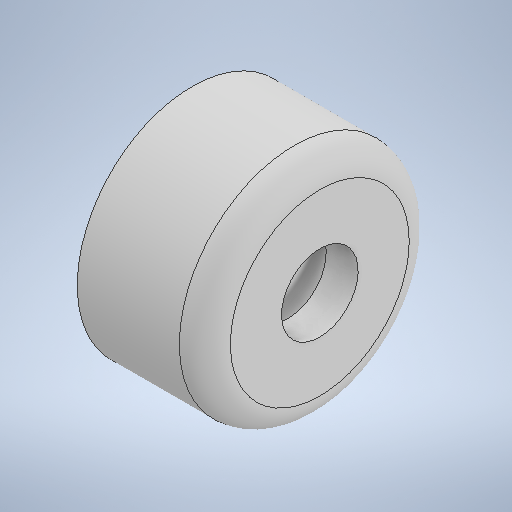
# Autodesk Inventor part: 14.2
Saved by Autodesk Inventor 2025.1 (Build 291241000, 241)
## iProperties
Created: 2024-09-13
Part Number: 14.2
Material: Generisch
Document SubType Name: Modeling
Designer: ffogue
Density: 1 g/cm^3
Appearance: Vorgabe
Author: ffogue
Autodesk Inventor part; units mm, degrees
ref_plane "YZ Plane" through (0, 0, 0) normal (1, 0, 0) x (0, 1, 0)
ref_plane "XZ Plane" through (0, 0, 0) normal (0, 1, 0) x (-1, 0, 0)
ref_plane "XY Plane" through (0, 0, 0) normal (0, 0, 1) x (1, 0, 0)
sketch "Sketch1" plane through (0, 0, 0) normal (0, 0, 1) x (1, 0, 0)
  line L0 (0, 6) -> (0, 9)
  line L1 (0, 9) -> (10, 9)
  line L2 (10, 9) -> (10, 0)
  line L3 (10, 0) -> (0, 0)
  line L4 (0, 6) -> (5.5, 6)
  line L5 (5.5, 6) -> (7.5, 4)
  line L6 (7.5, 4) -> (7.5, 0)
  point P0 (5, 9)
  dimension "d0" = 45
  dimension "d1" = 18
  dimension "d2" = 12
  dimension "d3" = 2.5
  dimension "d4" = 10
  dimension "d5" = 2
  constraints: 14 end point, 4 perpendicular, 1 horizontal, 1 midpoint, 1 point on line, 1 vertical, 1 vertical alignment
  measures "d0" angle of L5 L4
  measures "d1" diameter of point (5, 9) L3
  measures "d2" diameter of L4 L3
  measures "d3" distance between parallel lines of L2 L6
  measures "d4" distance of L0.end L1.end
  measures "d5" distance from line of L5.end L4
revolve "Revolution1" add sketch "Sketch1" angle 360 about axis through (10, 0, 0) along (-1, 0, 0)
thread "Thread1" size "M12x1.75" class "6H" standard "ISO Metric profile" full length
sketch "Sketch2" plane through (10, 0, 0) normal (1, 0, 0) x (0, 0, -1)
  circle A0 centre (0, 0) radius 9 projected
  constraints: 1 coincident
hole "Hole1" at (10, 0, 0) direction (-1, 0, 0) diameter 6 end through all
fillet "Fillet1" radius 2 1 edges at (10, -9, 0)
body "Solid1"
